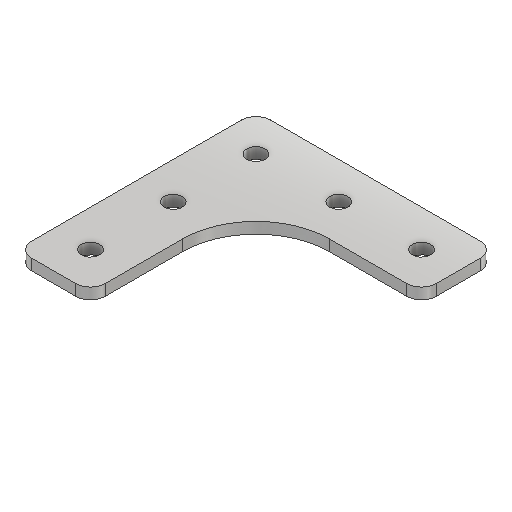
# Autodesk Inventor part: LC_ALU_3mm_Top_Beam_Mounting_Bracket
Saved by Autodesk Inventor 2026.1 (Build 301233000, 233)
## iProperties
Created: 2017-05-23
Part Number: LC_ALU_3mm_Top_Beam_Mounting_Bracket
Material: Aluminium 6061-AHC
Document SubType Name: Modeling
Designer: Andrzej
Density: 2.7 g/cm^3
Appearance: Aluminium - polerowane
Mass: 17.581 g
Surface Area: 53.0511 cm^2
Volume: 6.51149 cm^3
Author: Andrzej
Autodesk Inventor part; units mm, degrees
ref_plane "YZ Plane" through (0, 0, 0) normal (1, 0, 0) x (0, 1, 0)
ref_plane "XZ Plane" through (0, 0, 0) normal (0, 1, 0) x (-1, 0, 0)
ref_plane "XY Plane" through (0, 0, 0) normal (0, 0, 1) x (1, 0, 0)
sketch "Szkic1" plane through (0, 0, 0) normal (0, 0, 1) x (1, 0, 0)
  line L0 (-9.6941, 6.7253) -> (-9.6941, -58.2747)
  line L1 (-9.6941, 6.7253) -> (55.3059, 6.7253)
  line L2 (55.3059, 6.7253) -> (55.3059, -13.2747)
  line L3 (55.3059, -13.2747) -> (10.3059, -13.2747)
  line L4 (10.3059, -13.2747) -> (10.3059, -58.2747)
  line L5 (10.3059, -58.2747) -> (-9.6941, -58.2747)
  point P0 (0, 0)
  point P1 (0.3059, -48.2747)
  point P2 (0.3059, -25.7747)
  point P3 (0.3059, -3.2747)
  point P4 (45.3059, -3.2747)
  point P5 (22.8059, -3.2747)
  dimension "d0" = 65
  dimension "d1" = 65
  dimension "d2" = 20
  dimension "d4" = 10
  dimension "d5" = 10
  dimension "d6" = 20
  dimension "d7" = 10
  dimension "d8" = 10
  dimension "d9" = 10
  dimension "d10" = 22.5
  dimension "d11" = 22.5
  dimension "d12" = 10
  dimension "d13" = 10
  dimension "d14" = 10
  constraints: 12 end point, 4 perpendicular, 1 horizontal, 1 vertical
  measures "d0" distance of L0.start L0.end
  measures "d1" distance of L0.start L1.end
  measures "d2" distance of L1.end L2.end
  measures "d4" distance from line of L5 point (0.306, -48.275)
  measures "d5" distance from line of L0 point (0.306, -48.275)
  measures "d6" distance of L4.end L0.end
  measures "d7" distance from line of L0 point (0.306, -3.275)
  measures "d8" distance from line of L1 point (0.306, -3.275)
  measures "d9" distance from line of L0 point (0.306, -25.775)
  measures "d10" distance of point (0.306, -3.275) point (0.306, -25.775)
  measures "d11" distance of point (22.806, -3.275) point (0.306, -3.275)
  measures "d12" distance from line of L1 point (22.806, -3.275)
  measures "d13" distance from line of L1 point (45.306, -3.275)
  measures "d14" distance from line of L2 point (45.306, -3.275)
extrude "Wyciągnięcie proste1" add sketch "Szkic1" along normal blind 3
hole "Otwór1" at (0.3059, -48.2747, 0) at (0.3059, -25.7747, 0) at (0.3059, -3.2747, 0) at (45.3059, -3.2747, 0) at (22.8059, -3.2747, 0) direction (0, 0, 1) diameter 5 end through all
fillet "Zaokrąglenie1" radius 4 5 edges at (-9.6941, 6.7253, 1.5) (55.3059, 6.7253, 1.5) (55.3059, -13.2747, 1.5) (10.3059, -58.2747, 1.5) (-9.6941, -58.2747, 1.5)
fillet "Zaokrąglenie2" radius 20 1 edges at (10.3059, -13.2747, 1.5)
equation "\"d11\" = d10"
